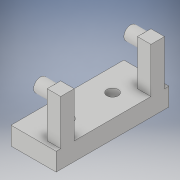
# Autodesk Inventor part: LaserMount
Saved by Autodesk Inventor 2019 (Build 230136000, 136)
## iProperties
Created: 2019-05-12
Part Number: LaserMount
Material: Generic
Document SubType Name: Modeling
Designer: Henry
Density: 1 g/cm^3
Appearance: Default
Author: Henry
Autodesk Inventor part; units mm, degrees
ref_plane "YZ Plane" through (0, 0, 0) normal (1, 0, 0) x (0, 1, 0)
ref_plane "XZ Plane" through (0, 0, 0) normal (0, 1, 0) x (-1, 0, 0)
ref_plane "XY Plane" through (0, 0, 0) normal (0, 0, 1) x (1, 0, 0)
sketch "Sketch1" plane through (0, 0, 0) normal (0, 1, 0) x (-1, 0, 0)
  line L0 (0, 0) -> (10, 0)
  line L1 (10, 0) -> (10, -25)
  line L2 (10, -25) -> (0, -25)
  line L3 (0, -25) -> (0, 0)
  dimension "d0" = 10
  dimension "d1" = 25
  constraints: 8 end point, 2 parallel, 1 horizontal, 1 perpendicular
  measures "d0" distance of L1.end L2.end
  measures "d1" distance of L0.end L1.end
extrude "Extrusion1" add sketch "Sketch1" along normal blind 4
sketch "Sketch2" plane through (0, 4, 0) normal (0, 1, 0) x (1, 0, 0)
  line L0 (0, 0) -> (0, 12.5)
  line L1 (0, 0) -> (0, 25) projected
  line L2 (0, 12.5) -> (0, 7.5)
  line L3 (0, 12.5) -> (0, 17.5)
  line L4 (0, 17.5) -> (-5, 17.5)
  line L5 (-10, 25) -> (-10, 0) projected
  circle A0 centre (-5, 17.5) radius 1.25
  line L6 (0, 7.5) -> (-5, 7.5)
  circle A1 centre (-5, 7.5) radius 1.25
  dimension "d4" = 12.5
  dimension "d5" = 5
  dimension "d6" = 5
  dimension "d7" = 5
  dimension "d8" = 2.5
  dimension "d9" = 5
  dimension "d10" = 2.5
  constraints: 10 end point, 2 centre point, 2 coincident, 2 point on line, 1 horizontal, 1 midpoint, 1 perpendicular
  measures "d4" distance of L0.start L0.end
  measures "d5" distance of L0.end L2.end
  measures "d6" distance of L0.end L3.end
  measures "d7" distance of L3.end L4.end
  measures "d8" diameter of A0
  measures "d9" distance of L2.end L6.end
  measures "d10" diameter of A1
extrude "Extrusion2" cut sketch "Sketch2" against normal blind 5
sketch "Sketch3" plane through (0, 4, 0) normal (0, 1, 0) x (1, 0, 0)
  line L0 (0, 25) -> (0, 0) projected
  line L1 (0, 25) -> (0, 24)
  line L2 (0, 24) -> (-3, 24)
  line L3 (-3, 24) -> (-3, 21)
  line L4 (-3, 21) -> (0, 21)
  line L5 (0, 21) -> (0, 24)
  line L6 (0, 0) -> (0, 1)
  line L7 (0, 1) -> (-3, 1)
  line L8 (-3, 1) -> (-3, 4)
  line L9 (-3, 4) -> (0, 4)
  line L10 (0, 4) -> (0, 1)
  dimension "d13" = 1
  dimension "d14" = 3
  dimension "d15" = 3
  dimension "d16" = 1
  dimension "d17" = 3
  dimension "d18" = 3
  constraints: 20 end point, 4 parallel, 2 horizontal, 2 perpendicular, 2 point on line
  measures "d13" distance of L0.start L1.end
  measures "d14" distance of L4.end L3.end
  measures "d15" distance of L3.end L2.end
  measures "d16" distance of L0.end L6.end
  measures "d17" distance of L8.end L9.end
  measures "d18" distance of L7.end L8.end
extrude "Extrusion3" add sketch "Sketch3" along normal blind 10
sketch "Sketch4" plane through (-3, 4, -24) normal (-1, 0, 0) x (0, 0, 1)
  line L0 (0, 0) -> (0, 10) projected
  line L1 (0, 10) -> (1.5, 10)
  line L2 (1.5, 10) -> (1.5, 8.5)
  line L3 (1.5, 8.5) -> (0, 8.5)
  line L4 (0, 8.5) -> (0, 10)
  circle A0 centre (1.5, 8.5) radius 1.5
  line L5 (23, 10) -> (20, 10) projected
  line L6 (23, 10) -> (21.5, 10)
  line L7 (21.5, 10) -> (21.5, 8.5)
  line L8 (21.5, 8.5) -> (23, 8.5)
  line L9 (23, 8.5) -> (23, 10)
  circle A1 centre (21.5, 8.5) radius 1.5
  point P0 (24, -4)
  dimension "d21" = 1.5
  dimension "d22" = 1.5
  dimension "d23" = 3
  dimension "d24" = 1.5
  dimension "d25" = 1.5
  dimension "d26" = 3
  constraints: 16 end point, 4 parallel, 2 centre point, 2 coincident, 2 horizontal, 2 perpendicular
  measures "d21" distance of L2.end L3.end
  measures "d22" distance of L1.end L2.end
  measures "d23" diameter of A0
  measures "d24" distance of L8.end L7.end
  measures "d25" distance of L7.end L6.end
  measures "d26" diameter of A1
extrude "Extrusion4" add sketch "Sketch4" along normal blind 3 contours A0 L2 L3 | L3 L2 A0 | A1 L8 L7 | L7 L8 A1
body "Solid1"
